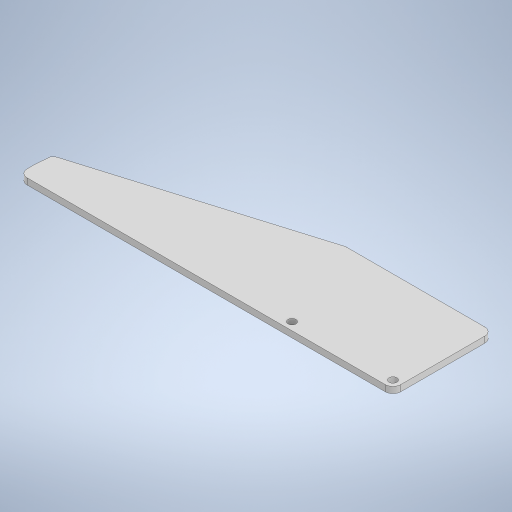
# Autodesk Inventor part: guideCam
Saved by Autodesk Inventor 2023 (Build 270158000, 158)
## iProperties
Created: 2022-09-15
Part Number: guideCam
Material: Generic
Document SubType Name: Modeling
Designer: deli
Density: 1 g/cm^3
Appearance: Default
Author: deli
Autodesk Inventor part; units mm, degrees
ref_plane "YZ Plane" through (0, 0, 0) normal (1, 0, 0) x (0, 1, 0)
ref_plane "XZ Plane" through (0, 0, 0) normal (0, 1, 0) x (-1, 0, 0)
ref_plane "XY Plane" through (0, 0, 0) normal (0, 0, 1) x (1, 0, 0)
sketch "Sketch1" plane through (0, 0, 0) normal (0, 1, 0) x (-1, 0, 0)
  arc A0 (186.6061, -4) -> (182.6061, 0) centre (182.6061, -4) ccw
  line L0 (0, 0) -> (182.6061, 0)
  arc A1 (0, 0) -> (-4, -4) centre (0, -4) ccw
  line L1 (-4, -46.8317) -> (-4, -4)
  arc A2 (-4, -46.8317) -> (0, -50.8317) centre (0, -46.8317) ccw
  line L2 (0, -50.8317) -> (70.4101, -50.8317)
  arc A3 (70.4101, -50.8317) -> (71.5648, -50.6614) centre (70.4101, -46.8317) ccw
  line L3 (71.5648, -50.6614) -> (183.7608, -16.8317)
  arc A4 (183.7608, -16.8317) -> (185.96, -15.1817) centre (182.6061, -13.002) ccw
  line L4 (186.6061, -8) -> (185.96, -15.1817)
  line L5 (186.6061, -4) -> (186.6061, -8)
  circle A5 centre (0, -4) radius 2
  circle A6 centre (51.4899, -4) radius 2
  constraints: 12 end point, 10 point on circle, 7 centre point
extrude "Extrusion1" add sketch "Sketch1" along normal blind 3.175
body "Solid1"
